board_controller (Autodesk Fusion 360 design; units mm, degrees)
Autodesk Fusion 360 part; units mm, degrees
sketch "Sketch1" plane through (0, 0, 0) normal (0, 1, 0) x (1, 0, 0)
  line L0 (0, 0) -> (-85, 0)
  line L1 (0, 0) -> (0, -98)
  line L2 (-85, 0) -> (-85, -20)
  line L3 (-85, -20) -> (-73, -20)
  line L4 (-73, -20) -> (-73, -68)
  line L5 (-73, -68) -> (-50, -98)
  line L6 (-50, -98) -> (0, -98)
  line L7 (50, -98) -> (0, -98)
  line L8 (73, -68) -> (50, -98)
  line L9 (73, -20) -> (73, -68)
  line L10 (85, -20) -> (73, -20)
  line L11 (85, 0) -> (85, -20)
  line L12 (0, 0) -> (85, 0)
  dimension "d1" = 85
  dimension "d2" = 20
  dimension "d3" = 12
  dimension "d4" = 48
  dimension "d5" = 98
  dimension "d6" = 50
  constraint coincident L0.start L1.start
  constraint horizontal L0
  constraint perpendicular L0 L1
  constraint perpendicular L0 L2
  constraint perpendicular L2 L3
  constraint perpendicular L3 L4
  constraint coincident L1 L6.end
  constraint perpendicular L1 L6
  constraint coincident L1.end L6
  constraint symmetric L0.start L1 L12.start
  constraint symmetric L0.end L1 L11.start
  constraint symmetric L1 L2.end L10.start
  constraint symmetric L1 L3.end L9.start
  constraint symmetric L1 L4.end L8.start
  constraint symmetric L1 L5.end L7.start
  constraint symmetric L1 L6.end L7.end
  measures "d1" distance of L0.start L0.end
  measures "d2" distance of L0.end L2.end
  measures "d3" distance of L2.end L3.end
  measures "d4" distance of L3.end L4.end
  measures "d5" distance of L0 L6
  measures "d6" distance of L5.end L1.end
extrude "Extrude1" add sketch "Sketch1" along normal blind 10
sketch "Sketch2" plane through (0, 10, 0) normal (0, 1, 0) x (-1, 0, 0)
  line L0 (85, 0) -> (85, 20)
  line L1 (85, 20) -> (73, 20)
  line L2 (73, 20) -> (73, 68)
  line L3 (73, 68) -> (50, 98)
  line L4 (50, 98) -> (-50, 98)
  line L5 (-50, 98) -> (-73, 68)
  line L6 (-73, 68) -> (-73, 20)
  line L7 (-73, 20) -> (-85, 20)
  line L8 (-85, 20) -> (-85, 0)
  line L9 (-85, 0) -> (85, 0)
  line L10 (-63, 0) -> (-63, 64.6078)
  line L11 (-63, 64.6078) -> (-37.3993, 98)
  line L12 (0, 98) -> (0, 0)
  line L13 (63, 64.6078) -> (37.3993, 98)
  line L14 (63, 0) -> (63, 64.6078)
  dimension "d9" = 10
  dimension "d10" = 10
  constraint coincident L9 L10.start
  constraint perpendicular L9 L10
  constraint coincident L4 L11.end
  constraint parallel L5 L11
  constraint midpoint L4 L12.start
  constraint coincident L12.end origin
  constraint symmetric L10.start L12 L14.start
  constraint symmetric L10.end L12 L13.start
  constraint symmetric L11.end L12 L13.end
  measures "d9" distance of L6 L10
  measures "d10" distance of L5 L11
extrude "Extrude2" add sketch "Sketch2" along normal blind 21.5 contours L4 L9 L12 L13 L14 | L4 L9 L10 L11 L12
sketch "Sketch3" plane through (0, 10, 0) normal (0, 1, 0) x (-1, 0, 0)
  line L0 (-63, 64.6078) -> (-37.3993, 98)
  line L1 (-37.3993, 98) -> (-50, 98)
  line L2 (-50, 98) -> (-73, 68)
  line L3 (-73, 68) -> (-73, 20)
  line L4 (-73, 20) -> (-85, 20)
  line L5 (-85, 20) -> (-85, 0)
  line L6 (-85, 0) -> (-63, 0)
  line L7 (-63, 0) -> (-63, 64.6078)
  line L8 (-73, 20) -> (-85, 20)
  line L9 (-85, 20) -> (-85, 0)
  line L10 (-85, 0) -> (-73, 0)
  line L11 (-73, 0) -> (-73, 20)
  line L12 (0, 0) -> (0, 105.5931)
  line L13 (73, 20) -> (85, 20)
  line L14 (73, 0) -> (73, 20)
  line L15 (85, 20) -> (85, 0)
  line L16 (85, 0) -> (73, 0)
  line L17 (-68.17, 74.3) -> (-60.2339, 68.2157)
  line L18 (-60.2339, 68.2157) -> (-63, 64.6078)
  line L19 (-63, 60) -> (-73, 60)
  line L20 (-73, 68) -> (-68.17, 74.3)
  line L21 (-73, 68) -> (-73, 60)
  line L22 (-63, 60) -> (-63, 64.6078)
  line L23 (63, 60) -> (73, 60)
  line L24 (63, 60) -> (63, 64.6078)
  line L25 (60.2339, 68.2157) -> (63, 64.6078)
  line L26 (68.17, 74.3) -> (60.2339, 68.2157)
  line L27 (73, 68) -> (68.17, 74.3)
  line L28 (73, 68) -> (73, 60)
  dimension "d15" = 8
  dimension "d20" = 6.3
  constraint horizontal L8
  constraint vertical L9
  constraint horizontal L10
  constraint vertical L11
  constraint coincident L5.end L6.start
  constraint coincident L3.end L4.start
  constraint coincident L12.start origin
  constraint vertical L12
  constraint symmetric L3.end L12 L13.start
  constraint symmetric L4.end L12 L13.end
  constraint symmetric L5.end L12 L15.end
  constraint symmetric L10.end L12 L14.start
  constraint coincident L2 L17.start
  constraint coincident L0 L17.end
  constraint perpendicular L0 L17
  constraint coincident L0.start L7.end
  constraint coincident L7 L19.start
  constraint coincident L3 L19.end
  constraint perpendicular L3 L19
  constraint coincident L2.end L3.start
  constraint symmetric L12 L17.start L26.start
  constraint symmetric L12 L17.end L25.start
  constraint symmetric L12 L0.start L24.end
  constraint symmetric L12 L19.start L23.start
  constraint symmetric L12 L19.end L23.end
  constraint symmetric L12 L2.end L27.start
  measures "d15" distance of L19.end L2.end
  measures "d20" vertical distance of L17.start L2.end
extrude "Extrude3" cut sketch "Sketch3" against normal blind 6.5 contours L0 L2 L3 L7 L17 L18 L19 L20 L21 L22 | L4 L5 L6 L8 L9 L10 L11 | L13 L14 L15 L16 | L23 L24 L25 L26 L27 L28
equation "d1 = ( 170 / 2 ) * 1 mm"
equation "d10 = d9"
